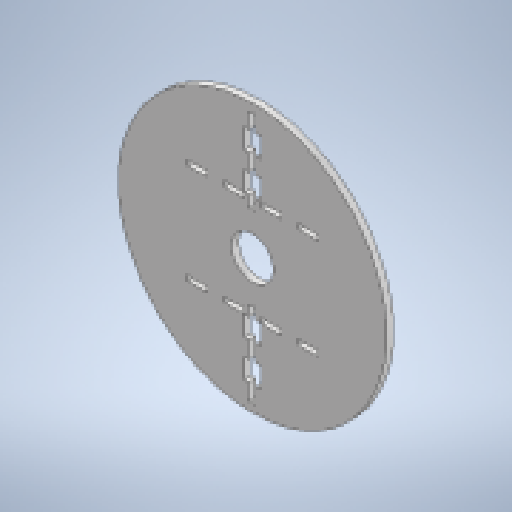
# Autodesk Inventor part: лицо1
Saved by Autodesk Inventor 2023 (Build 270158000, 158)
## iProperties
Created: 2024-12-06
Part Number: лицо1
Material: Типовые
Document SubType Name: Modeling
Designer: DELL
Density: 1 g/cm^3
Appearance: По умолчанию
Author: DELL
Autodesk Inventor part; units mm, degrees
ref_plane "YZ Plane" through (0, 0, 0) normal (1, 0, 0) x (0, 1, 0)
ref_plane "XZ Plane" through (0, 0, 0) normal (0, 1, 0) x (-1, 0, 0)
ref_plane "XY Plane" through (0, 0, 0) normal (0, 0, 1) x (1, 0, 0)
sketch "Эскиз1" plane through (0, 0, 0) normal (0, 0, 1) x (1, 0, 0)
  circle A0 centre (0, 0) radius 80 projected
  line L0 (-52.7251, -56.1362) -> (-52.7358, -38.0942) construction
  arc A1 (-51.7364, -37.0936) -> (-52.7358, -38.0942) centre (-51.7358, -38.0936) ccw construction
  line L1 (-51.7364, -37.0936) -> (-13.2571, -37.0709) construction
  arc A2 (-12.2565, -38.0703) -> (-13.2571, -37.0709) centre (-13.2565, -38.0709) ccw construction
  line L2 (-12.2565, -38.0703) -> (-12.2459, -56.1122) construction
  arc A3 (-13.2453, -57.1128) -> (-12.2459, -56.1122) centre (-13.2459, -56.1128) ccw construction
  line L3 (-13.2453, -57.1128) -> (-51.7245, -57.1356) construction
  arc A4 (-52.7251, -56.1362) -> (-51.7245, -57.1356) centre (-51.7251, -56.1356) ccw construction
  circle A5 centre (-11.4805, -27.7164) radius 3.15 construction
  circle A6 centre (-27.7164, 11.4805) radius 3.15 construction
  circle A7 centre (11.4805, 27.7164) radius 3.15 construction
  circle A8 centre (27.7164, -11.4805) radius 3.15 construction
  circle A9 centre (0, 0) radius 12.5
  circle A10 centre (0, 0) radius 39.5 construction
  point P0 (0, 0)
  dimension "d10" = 25
  constraints: 1 centre point
  measures "d10" diameter of A9
extrude "Выдавливание1" add sketch "Эскиз1" along normal blind 4
sketch "Эскиз2" plane through (0, 0, 0) normal (0, 0, -1) x (-1, 0, 0)
  circle A0 centre (0, 0) radius 80 projected
  line L0 (0, 80) -> (0, -80) construction
  line L1 (2, -75) -> (-2, -75)
  line L2 (-2, -75) -> (-2, 75)
  line L3 (-2, 75) -> (2, 75)
  line L4 (2, 75) -> (2, -75)
  line L5 (2, -75) -> (-2, 75) construction
  line L6 (-2, -75) -> (2, 75) construction
  line L7 (-2, 25) -> (2, 25)
  line L8 (-2, -25) -> (2, -25)
  point P0 (0, -25)
  point P1 (0, 75)
  point P2 (0, 25)
  dimension "d2" = 4
  dimension "d3" = 150
  dimension "d4" = 50
  dimension "d5" = 50
  constraints: 18 end point, 5 midpoint, 4 point on line, 3 perpendicular, 2 parallel, 2 point on circle, 1 horizontal, 1 vertical
  measures "d2" distance of L2.end L3.end
  measures "d3" distance of L1.end L2.end
  measures "d4" distance from line of L1 point (0, -25)
  measures "d5" distance of point (0, 75) point (0, 25)
extrude "Выдавливание2" cut sketch "Эскиз2" against normal blind 10 contours L1 L2 L8 L4 | L7 L2 L3 L4
sketch "Эскиз3" plane through (0, 0, 4) normal (0, 0, 1) x (1, 0, 0)
  line L0 (5, 53.408) -> (2, 53.408)
  line L1 (2, 31.408) -> (2, 43.408)
  line L2 (17, 28.408) -> (5, 28.408)
  line L3 (39.1243, 28.408) -> (27, 28.408)
  line L4 (2, 53.408) -> (2, 65.4106)
  line L5 (5, 65.4106) -> (5, 53.408)
  line L6 (2, 65.4106) -> (5, 65.4106)
  line L7 (2, 43.408) -> (5, 43.408)
  line L8 (5, 31.408) -> (2, 31.408)
  line L9 (5, 43.408) -> (5, 31.408)
  line L10 (5, 28.408) -> (5, 31.408)
  line L11 (5, 31.408) -> (17, 31.408)
  line L12 (27, 31.408) -> (38.9975, 31.408)
  line L13 (38.9975, 31.408) -> (39.1243, 28.408)
  line L14 (17, 31.408) -> (17, 28.408)
  line L15 (27, 28.408) -> (27, 31.408)
  line L16 (5, 65.4121) -> (5, 65.4106)
  line L17 (102, 0) -> (-112, 0) construction
  line L18 (5, -53.408) -> (2, -53.408)
  line L19 (2, -31.408) -> (2, -43.408)
  line L20 (17, -28.408) -> (5, -28.408)
  line L21 (39.1243, -28.408) -> (27, -28.408)
  line L22 (2, -53.408) -> (2, -65.4106)
  line L23 (5, -65.4106) -> (5, -53.408)
  line L24 (2, -65.4106) -> (5, -65.4106)
  line L25 (2, -43.408) -> (5, -43.408)
  line L26 (5, -31.408) -> (2, -31.408)
  line L27 (5, -43.408) -> (5, -31.408)
  line L28 (5, -28.408) -> (5, -31.408)
  line L29 (5, -31.408) -> (17, -31.408)
  line L30 (27, -31.408) -> (38.9975, -31.408)
  line L31 (38.9975, -31.408) -> (39.1243, -28.408)
  line L32 (17, -31.408) -> (17, -28.408)
  line L33 (27, -28.408) -> (27, -31.408)
  line L34 (5, -65.4121) -> (5, -65.4106)
  line L35 (0, 116) -> (0, -113) construction
  line L36 (-5, 53.408) -> (-2, 53.408)
  line L37 (-2, 31.408) -> (-2, 43.408)
  line L38 (-17, 28.408) -> (-5, 28.408)
  line L39 (-39.1243, 28.408) -> (-27, 28.408)
  line L40 (-2, 53.408) -> (-2, 65.4106)
  line L41 (-5, 65.4106) -> (-5, 53.408)
  line L42 (-2, 65.4106) -> (-5, 65.4106)
  line L43 (-2, 43.408) -> (-5, 43.408)
  line L44 (-5, 31.408) -> (-2, 31.408)
  line L45 (-5, 43.408) -> (-5, 31.408)
  line L46 (-5, 28.408) -> (-5, 31.408)
  line L47 (-5, 31.408) -> (-17, 31.408)
  line L48 (-27, 31.408) -> (-38.9975, 31.408)
  line L49 (-38.9975, 31.408) -> (-39.1243, 28.408)
  line L50 (-17, 31.408) -> (-17, 28.408)
  line L51 (-27, 28.408) -> (-27, 31.408)
  line L52 (-5, 65.4121) -> (-5, 65.4106)
  line L53 (-17, -31.408) -> (-17, -28.408)
  line L54 (-17, -28.408) -> (-5, -28.408)
  line L55 (-5, -28.408) -> (-5, -31.408)
  line L56 (-5, -31.408) -> (-17, -31.408)
  line L57 (-5, -31.408) -> (-2, -31.408)
  line L58 (-5, -43.408) -> (-5, -31.408)
  line L59 (-2, -31.408) -> (-2, -43.408)
  line L60 (-2, -43.408) -> (-5, -43.408)
  line L61 (-5, -53.408) -> (-2, -53.408)
  line L62 (-5, -65.4106) -> (-5, -53.408)
  line L63 (-5, -65.4121) -> (-5, -65.4106)
  line L64 (-2, -53.408) -> (-2, -65.4106)
  line L65 (-2, -65.4106) -> (-5, -65.4106)
  line L66 (-27, -28.408) -> (-27, -31.408)
  line L67 (-27, -31.408) -> (-38.9975, -31.408)
  line L68 (-38.9975, -31.408) -> (-39.1243, -28.408)
  line L69 (-39.1243, -28.408) -> (-27, -28.408)
  point P0 (0, 0)
  constraints: 140 end point, 48 symmetric about line, 1 horizontal, 1 vertical
extrude "Выдавливание3" cut sketch "Эскиз3" against normal blind 10
